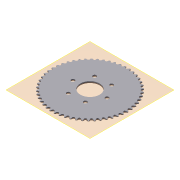
# Autodesk Inventor part: 25 sprocket 54T
Saved by Autodesk Inventor 2011 (Build 150239000, 239)
## iProperties
Created: 2011-07-16
Part Number: 25 sprocket 54T
Material: Aluminum-6061
Document SubType Name: Modeling
Designer: Dan Niemitalo
Density: 2.71 g/cm^3
Mass: 52.4276 g
Surface Area: 185.116 cm^2
Volume: 19.346 cm^3
CustomPartVersion: 1
Author: Dan Niemitalo
Autodesk Inventor part; units mm, degrees
ref_plane "YZ Plane" through (0, 0, 0) normal (1, 0, 0) x (0, 1, 0)
ref_plane "XZ Plane" through (0, 0, 0) normal (0, 1, 0) x (-1, 0, 0)
sketch "Theoretical Tooth Profile" plane through (0, 0, 0) normal (0, 0, 1) x (1, 0, 0)
  circle A0 centre (0, 0) radius 54.605 construction
  line L0 (0, 0) -> (0, 54.605) construction
  line L1 (0, 0) -> (6.3393, 54.2358) construction
  circle A1 centre (0, 0) radius 56.4176
  arc A2 (-1.3713, 53.6047) -> (1.3713, 53.6047) centre (0, 54.605) ccw
  line L2 (0, 54.605) -> (6.3393, 54.2358) construction
  line L3 (0, 54.605) -> (2.1341, 56.1619) construction
  line L4 (2.1341, 56.1619) -> (-1.9648, 54.7386) construction
  arc A3 (2.9062, 56.3427) -> (2.1253, 55.2007) centre (4.615, 54.3362) ccw
  arc A4 (-2.1253, 55.2007) -> (-2.9062, 56.3427) centre (-4.615, 54.3362) ccw
  line L5 (-4.615, 54.3362) -> (-2.1253, 55.2007) construction
  arc A5 (-1.9648, 54.7386) -> (-1.3713, 53.6047) centre (2.1341, 56.1619) ccw
  line L6 (-1.9648, 54.7386) -> (-2.1253, 55.2007)
  arc A6 (1.3713, 53.6047) -> (1.9648, 54.7386) centre (-2.1341, 56.1619) ccw
  line L7 (2.1253, 55.2007) -> (1.9648, 54.7386)
  line L8 (0, 0) -> (3.2804, 56.3222) construction
  point P0 (3.1696, 54.4204)
  dimension "d0" = 109.2101
  dimension "d2" = 6.667
  dimension "d3" = 1.6973
  dimension "d10" = 126.111
  dimension "d11" = 16.963
  dimension "d12" = 2.6416
  dimension "d13" = 4.339
  dimension "d14" = 4.6228
  dimension "d23" = 1.905
  constraints: 18 end point, 15 point on circle, 7 centre point, 3 coincident, 3 point on line, 3 symmetric about line, 3 tangent, 1 equal radius, 1 midpoint, 1 parallel, 1 vertical, 1 other
  measures "d0" diameter of A0
  measures "d2" angle of L1 L0
  measures "d3" radius of A2
  measures "d10" angle of L3 L0
  measures "d11" angle of L4 L3
  measures "d12" distance of L2.start L3.end
  measures "d13" distance of L3.end L4.end
  measures "d14" distance of A3.centre L0.end
  measures "d23" distance from line of L8.end L2
sketch "Tooth Profile" plane through (0, 0, 0) normal (0, 0, 1) x (1, 0, 0)
  circle A0 centre (0, 0) radius 56.4176 projected
  line L0 (0, 0) -> (0, 54.605) construction
  line L1 (0, 54.605) -> (1.5819, 53.9898) construction
  arc A1 (-1.5819, 53.9898) -> (1.5819, 53.9898) centre (0, 54.605) ccw
  line L2 (-1.5819, 53.9898) -> (0, 54.605) construction
  arc A2 (-1.5819, 53.9898) -> (-2.747, 56.3507) centre (-15.6153, 48.5326) ccw
  arc A3 (2.747, 56.3507) -> (1.5819, 53.9898) centre (15.6153, 48.5326) ccw
  dimension "d44" = 137.5
  dimension "d45" = 1.6973
  dimension "d46" = 15.0571
  constraints: 8 point on circle, 7 end point, 3 centre point, 2 tangent, 1 coincident, 1 equal radius, 1 symmetric about line, 1 vertical
  measures "d44" angle of L1 L2
  measures "d45" radius of A1
  measures "d46" radius of A3
sketch "Section Profile" plane through (0, 0, 0) normal (1, 0, 0) x (0, 1, 0)
  line L0 (56.4176, 0) -> (-56.4176, 0) projected
  line L1 (32.4804, 1.143) -> (-32.4804, 1.143)
  line L2 (-32.4804, 1.143) -> (-32.4804, -1.143)
  line L3 (-32.4804, -1.143) -> (32.4804, -1.143)
  line L4 (32.4804, -1.143) -> (32.4804, 1.143)
  line L5 (32.4804, 1.143) -> (56.4176, 1.143) construction
  line L6 (56.4176, 1.143) -> (56.4176, -1.143) construction
  line L7 (56.4176, -1.143) -> (32.4804, -1.143) construction
  line L8 (32.4804, -1.143) -> (32.4804, 1.143)
  arc A0 (56.4176, 0.3492) -> (53.2419, 1.143) centre (53.2419, -5.6071) ccw
  arc A1 (53.2419, -1.143) -> (56.4176, -0.3492) centre (53.2419, 5.6071) ccw
  line L9 (53.2419, 1.143) -> (0, 1.143)
  line L10 (0, 1.143) -> (0, -1.143)
  line L11 (0, -1.143) -> (53.2419, -1.143)
  line L12 (0, 1.143) -> (0, -1.143)
  line L13 (56.4176, 0.3492) -> (56.4176, -0.3492)
  point P0 (0, 0)
  point P1 (0, 0)
  dimension "d30" = 2.286
  dimension "d31" = 64.9608
  dimension "d32" = 2.286
  dimension "d33" = 0.7937
  dimension "d34" = 6.75
  dimension "d43" = 1.143
  constraints: 26 end point, 7 midpoint, 5 perpendicular, 4 parallel, 4 point on circle, 3 point on line, 3 symmetric about line, 2 centre point, 2 horizontal, 2 tangent, 1 collinear, 1 other
  measures "d30" distance between parallel lines of L7 L5
  measures "d31" distance between parallel lines of L2 L4
  measures "d32" distance between parallel lines of L3 L1
  measures "d33" distance from line of L13.start L5
  measures "d34" radius of A0
  measures "d43" distance between parallel lines of L3 L0
revolve "Shroud" add sketch "Section Profile" angle 360 about axis through (0, 0, 1.143) along (0, 0, -1) contours L10 L3 L2 L0 | L0 L2 L1 L10
revolve "Strand" add sketch "Section Profile" angle 360 about axis through (0, 0, 1.143) along (0, 0, -1) contours L13 A1 L11 L4 L0 | L0 L4 L9 A0 L13 | L4 L3 L10 L0 | L0 L10 L1 L4
pattern_of_one "Strand Pattern"
extrude "Theoretical Tooth" cut sketch "Theoretical Tooth Profile" along normal through all both and the other way through all contours A3 L7 A6 A2 A5 L6 A4 A1 picked at (0.323, 54.7781)
extrude "Tooth" [suppressed]
pattern_circular "Tooth Pattern" count 54 over 360 about axis through (0, 0, -10) along (0, 0, 1) of "Theoretical Tooth"
ref_plane "Timing Plane" through (0, 54.605, 0) normal (1, 0, 0) x (0, 1, 0)
sketch "Sketch4" plane through (0, 0, 1.143) normal (0, 0, 1) x (1, 0, 0)
  circle A0 centre (0, 0) radius 14.2812
  point P0 (0, 0)
  dimension "d67" = 28.5623
  constraints: 1 centre point, 1 coincident
  measures "d67" diameter of A0
extrude "Extrusion4" cut sketch "Sketch4" against normal through all
sketch "Sketch6" plane through (0, 0, 1.143) normal (0, 0, 1) x (0.8936326, -0.4487992, 0)
  circle A0 centre (0, 0) radius 23.8125 construction
  circle A1 centre (0, 23.8125) radius 2.6162
  circle A2 centre (-20.6222, 11.9063) radius 2.6162
  circle A3 centre (-20.6222, -11.9062) radius 2.6162
  circle A4 centre (0, -23.8125) radius 2.6162
  circle A5 centre (20.6222, -11.9063) radius 2.6162
  circle A6 centre (20.6222, 11.9062) radius 2.6162
  point P0 (0, 0)
  dimension "d68" = 47.625
  dimension "d69" = 5.2324
  dimension "d72" = 360
  constraints: 6 centre point, 2 coincident, 1 vertical alignment, 15 other
  measures "d69" diameter of A1
hole "Hole2" at (10.687, 21.2796, 1.143) at (23.7722, 1.3846, 1.143) at (13.0852, -19.8951, 1.143) at (-10.687, -21.2796, 1.143) at (-23.7722, -1.3846, 1.143) at (-13.0852, 19.8951, 1.143) direction (0, 0, -1) diameter 5.2324 end through all
equation "\"d3\" = 0.5 * da_Dr + da_SC"
equation "\"d12\" = 0.8 * da_Dr"
equation "\"d13\" = 1.3 * da_Dr + da_SC"
equation "\"d14\" = 1.4 * da_Dr"
equation "\"d23\" = da_Ha"
equation "\"d44\" = da_Alfa"
equation "\"d45\" = da_Ri"
equation "\"d46\" = da_Re"
equation "\"d30\" = da_Bf"
equation "\"d31\" = da_Ds"
equation "\"d32\" = da_Bs"
equation "\"d33\" = da_Ba"
equation "\"d34\" = da_Rx"
equation "\"d40\" = da_pt"
equation "\"form_type\" = 0"
equation "\"da_p\" = 6.35"
equation "\"da_Dr\" = 3.302"
equation "\"da_SC\" = 0.04636"
equation "\"da_Ha\" = 1.905"
equation "\"da_pt\" = 6.4008"
equation "\"da_Bf\" = 2.286"
equation "\"da_Ba\" = 0.79375"
equation "\"da_Rx\" = 6.75005"
equation "\"da_Ra\" = 0.254"
equation "\"da_Bs\" = 2.286"
equation "\"da_Ds\" = 64.96083"
equation "\"da_Re\" = 15.05712"
equation "\"da_Ri\" = 1.69735"
equation "\"da_Alfa\" = 137.5deg"
body "Solid1"
